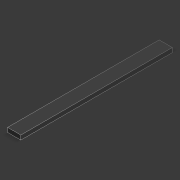
# Autodesk Inventor part: padding_strip
Saved by Autodesk Inventor 2020.2 (Build 242310000, 310)
## iProperties
Created: 2020-07-06
Part Number: padding_strip
Material: Rubber, Silicone
Document SubType Name: Modeling
Designer: isaac
Density: 1.25 g/cm^3
Appearance: Rubber - Black
Mass: 0.415826 g
Surface Area: 7.13621 cm^2
Volume: 0.415826 cm^3
Author: isaac
Autodesk Inventor part; units mm, degrees
ref_plane "YZ Plane" through (0, 0, 0) normal (1, 0, 0) x (0, 1, 0)
ref_plane "XZ Plane" through (0, 0, 0) normal (0, 1, 0) x (-1, 0, 0)
ref_plane "XY Plane" through (0, 0, 0) normal (0, 0, 1) x (1, 0, 0)
sketch "Sketch1" plane through (0, 0, 0) normal (0, 1, 0) x (-1, 0, 0)
  line L0 (0, 0) -> (4.7625, 0)
  line L1 (4.7625, 0) -> (4.7625, -54.625)
  line L2 (4.7625, -54.625) -> (0, -54.625)
  line L3 (0, -54.625) -> (0, 0)
  dimension "d0" = 4.7625
  dimension "d1" = 54.625
  constraints: 8 end point, 2 parallel, 1 horizontal, 1 perpendicular
  measures "d0" distance of L1.end L2.end
  measures "d1" distance of L0.end L1.end
extrude "Extrusion1" add sketch "Sketch1" along normal blind 1.5875
equation "\"d0\" = foamPadWidth"
equation "\"d1\" = overallLength"
equation "\"d2\" = foamPadThick"
equation "\"foamPadWidth\" = 4.7625"
equation "\"overallLength\" = 54.625"
equation "\"foamPadThick\" = 1.5875"
body "Solid1"
